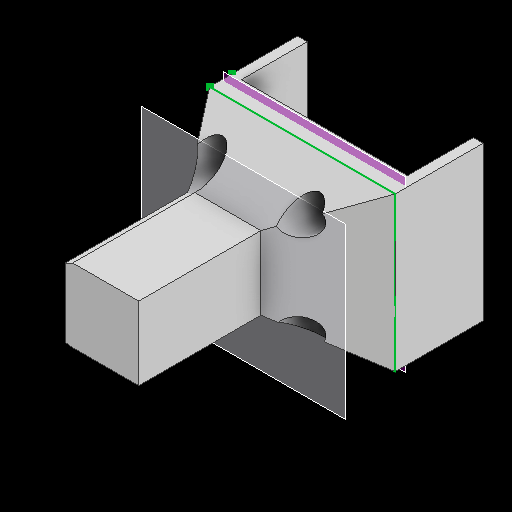
# Autodesk Inventor part: spring_connector
Saved by Autodesk Inventor 2025.1 (Build 291241000, 241)
## iProperties
Created: 2024-08-22
Part Number: spring_connector
Material: 일반
Document SubType Name: Modeling
Designer: ojs08
Density: 1 g/cm^3
Appearance: 기본값
Author: ojs08
Autodesk Inventor part; units mm, degrees
ref_plane "YZ Plane" through (0, 0, 0) normal (1, 0, 0) x (0, 1, 0)
ref_plane "XZ Plane" through (0, 0, 0) normal (0, 1, 0) x (-1, 0, 0)
ref_plane "XY Plane" through (0, 0, 0) normal (0, 0, 1) x (1, 0, 0)
sketch "스케치1" plane through (0, 0, 0) normal (0, 0, 1) x (1, 0, 0)
  line L0 (0, 0) -> (38, 0)
  line L1 (38, 0) -> (38, -31.5)
  line L2 (38, -31.5) -> (0, -31.5)
  line L3 (0, -31.5) -> (0, 0)
  dimension "d0" = 38
  dimension "d1" = 31.5
  constraints: 8 end point, 2 parallel, 1 coincident, 1 horizontal, 1 perpendicular
  measures "d0" distance of L1.end L2.end
  measures "d1" distance of L0.end L1.end
extrude "돌출1" add sketch "스케치1" along normal blind 18
sketch "스케치2" plane through (0, 0, 0) normal (0, 0, -1) x (-1, 0, 0)
  line L0 (0, -31.5) -> (-38, -31.5) projected
  line L1 (0, 0) -> (0, -31.5) projected
  line L2 (-38, 0) -> (0, 0) projected
  line L3 (-38, -31.5) -> (-38, 0) projected
  line L4 (-2, -31.5) -> (-2, 0)
  line L5 (0, -31.5) -> (-38, -31.5) projected
  line L6 (-36, -31.5) -> (-36, 0)
  dimension "d4" = 2
  dimension "d5" = 2
  constraints: 4 end point, 4 point on line, 2 perpendicular
  measures "d4" distance between parallel lines of L1 L4
  measures "d5" distance between parallel lines of L3 L6
extrude "돌출2" cut sketch "스케치2" against normal blind 13.5 contours L0 L6 L2 L4
sketch "스케치3" plane through (0, 0, 18) normal (0, 0, 1) x (1, 0, 0)
  point P0 (0, 0)
ref_plane "작업 평면1" through (0, 0, 30) normal (0, 0, 1) x (1, 0, 0)
sketch "스케치4" plane through (0, 0, 18) normal (0, 0, 1) x (1, 0, 0)
  line L0 (0, -31.5) -> (38, -31.5) projected
  line L1 (38, -31.5) -> (38, 0) projected
  line L2 (38, 0) -> (0, 0) projected
  line L3 (0, 0) -> (0, -31.5) projected
sketch "스케치5" plane through (0, 0, 30) normal (0, 0, 1) x (1, 0, 0)
  line L0 (0, 0) -> (0, -31.5) projected
  line L1 (0, -31.5) -> (38, -31.5) projected
  line L2 (7.5, -8.25) -> (22.5, -8.25)
  line L3 (22.5, -8.25) -> (22.5, -23.25)
  line L4 (22.5, -23.25) -> (7.5, -23.25)
  line L5 (7.5, -23.25) -> (7.5, -8.25)
  point P0 (15, -15.75)
  point P1 (15, -23.25)
  dimension "d9" = 15
  dimension "d10" = 15.75
  dimension "d11" = 15
  dimension "d12" = 15
  dimension "d13" = 7.5
  dimension "d14" = 7.5
  constraints: 8 end point, 2 parallel, 1 horizontal, 1 midpoint, 1 perpendicular
  measures "d9" distance from line of L0 point (15, -15.75)
  measures "d10" distance from line of L1 point (15, -15.75)
  measures "d11" distance of L2.start L2.end
  measures "d12" distance of L2.end L3.end
  measures "d13" distance from line of L3 point (15, -15.75)
  measures "d14" distance of point (15, -23.25) point (15, -15.75)
loft "로프트1" add profiles "스케치5" section 2 edges at (19, -31.5, 18) (38, -15.75, 18) (19, 0, 18) (0, -15.75, 18)
sketch "스케치6" plane through (0, 0, 13.5) normal (0, 0, -1) x (-1, 0, 0)
  line L0 (-2, -31.5) -> (-36, -31.5) projected
  line L1 (-2, 0) -> (-2, -31.5) projected
  line L2 (-36, 0) -> (-2, 0) projected
  line L3 (-36, -31.5) -> (-36, 0) projected
  circle A0 centre (-7, -26) radius 2
  circle A1 centre (-7, -6) radius 2
  circle A2 centre (-27, -26) radius 2
  circle A3 centre (-27, -6) radius 2
  point P0 (0, 0)
  dimension "d19" = 4
  dimension "d20" = 5
  dimension "d21" = 5.5
  dimension "d24" = 20
  dimension "d31" = 20
  constraints: 4 centre point, 1 horizontal, 1 vertical, 6 other
  measures "d19" diameter of A0
  measures "d20" distance from line of L1 A0.centre
  measures "d21" distance from line of L0 A0.centre
  measures "d24" distance of A0.centre A1.centre
  measures "d31" distance of A0.centre A2.centre
extrude "돌출3" cut sketch "스케치6" against normal blind 2 contours A0 | A1 | A2 | A3
sketch "스케치7" plane through (0, 0, 13.5) normal (0, 0, -1) x (-1, 0, 0)
  circle A0 centre (-7, -26) radius 2 projected
  circle A1 centre (-7, -6) radius 2 projected
  circle A2 centre (-27, -6) radius 2 projected
  circle A3 centre (-27, -26) radius 2 projected
  circle A4 centre (-7, -26) radius 2.7017
  point P0 (0, 0)
  constraints: 1 centre point
ref_plane "작업 평면2" through (0, 0, 15.5) normal (0, 0, -1) x (-1, 0, 0)
sketch "스케치8" plane through (0, 0, 13.5) normal (0, 0, -1) x (-1, 0, 0)
  circle A0 centre (-7, -26) radius 2.7017 projected
  circle A1 centre (-7, -26) radius 2 projected
  circle A2 centre (-7, -26) radius 3
  point P0 (0, 0)
  dimension "d39" = 0.7017
  dimension "d40" = 6
  constraints: 1 centre point, 1 concentric
  measures "d39" radial gap between concentric circles of A0 A1
  measures "d40" diameter of A2
sketch "스케치9" plane through (0, 0, 13.5) normal (0, 0, -1) x (-1, 0, 0)
  circle A0 centre (-7, -6) radius 3
  circle A1 centre (-27, -6) radius 3
  circle A2 centre (-27, -26) radius 3
  circle A3 centre (-27, -26) radius 2 projected
  circle A4 centre (-27, -6) radius 2 projected
  circle A5 centre (-7, -6) radius 2 projected
  point P0 (0, 0)
  dimension "d41" = 6
  dimension "d42" = 6
  dimension "d43" = 6
  constraints: 3 centre point, 3 concentric
  measures "d41" diameter of A0
  measures "d42" diameter of A1
  measures "d43" diameter of A2
sketch "스케치10" plane through (0, 0, 13.5) normal (0, 0, -1) x (-1, 0, 0)
  circle A0 centre (-7, -26) radius 3 projected
  circle A1 centre (-27, -26) radius 3 projected
  circle A2 centre (-27, -6) radius 3 projected
  circle A3 centre (-7, -6) radius 3 projected
  point P0 (0, 0)
extrude "돌출4" cut sketch "스케치8" against normal blind 16 from surface at -2 contours A0 | A1 | A2
extrude "돌출5" cut sketch "스케치9" against normal blind 16 from surface at -2 contours A2 | A3
extrude "돌출6" cut sketch "스케치10" against normal blind 16 from surface at -2 contours A3
sketch "스케치11" plane through (0, 0, 13.5) normal (0, 0, -1) x (-1, 0, 0)
  circle A0 centre (-27, -6) radius 3
  circle A1 centre (-27, -6) radius 2 projected
  point P0 (0, 0)
  dimension "d50" = 6
  constraints: 1 centre point, 1 concentric
  measures "d50" diameter of A0
extrude "돌출7" cut sketch "스케치11" against normal blind 16 from surface at -2 contours A0 | A1
sketch "스케치12" plane through (0, 0, 30) normal (0, 0, 1) x (1, 0, 0)
  arc A0 (7.5, -8.958) -> (8.9843, -8.25) centre (7, -6) ccw projected
  line L0 (7.5, -23.042) -> (7.5, -8.958) projected
  arc A1 (8.199, -23.25) -> (7.5, -23.042) centre (7, -26) ccw projected
  line L1 (22.5, -23.25) -> (8.199, -23.25) projected
  line L2 (22.5, -8.25) -> (22.5, -23.25) projected
  line L3 (8.9843, -8.25) -> (22.5, -8.25) projected
  point P0 (0, 0)
extrude "돌출8" add sketch "스케치12" along normal blind 25
sketch "스케치13" plane through (8.199, -23.25, 30) normal (0, -1, 0) x (1, 0, 0)
  circle A0 centre (6.801, 18.85) radius 4.25
  line L0 (14.301, 0) -> (0, 0) projected
  line L1 (14.301, 0) -> (14.301, 25) projected
  point P0 (-8.199, -30)
  dimension "d55" = 18.85
  dimension "d56" = 7.5
  dimension "d57" = 8.5
  constraints: 1 centre point
  measures "d55" distance from line of A0.centre L0
  measures "d56" distance from line of L1 A0.centre
  measures "d57" diameter of A0
extrude "돌출9" cut sketch "스케치13" against normal blind 3
